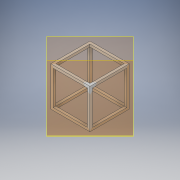
# Autodesk Inventor part: Outer
Saved by Autodesk Inventor 2019 (Build 230136000, 136)
## iProperties
Created: 2019-05-01
Part Number: Outer
Material: Generic
Document SubType Name: Modeling
Designer: Jorian Brusind
Density: 1 g/cm^3
Appearance: Default
Author: Jorian Brusind
Autodesk Inventor part; units mm, degrees
ref_plane "YZ Plane" through (0, 0, 0) normal (1, 0, 0) x (0, 1, 0)
ref_plane "XZ Plane" through (0, 0, 0) normal (0, 1, 0) x (-1, 0, 0)
ref_plane "XY Plane" through (0, 0, 0) normal (0, 0, 1) x (1, 0, 0)
sketch "Sketch1" plane through (0, 0, 0) normal (0, 1, 0) x (-1, 0, 0)
  line L0 (0, 0) -> (15, 0)
  line L1 (15, 0) -> (15, -15)
  line L2 (15, -15) -> (0, -15)
  line L3 (0, -15) -> (0, 0)
  dimension "d0" = 15
  dimension "d1" = 15
  constraints: 8 end point, 2 parallel, 1 horizontal, 1 perpendicular
  measures "d0" distance of L1.end L2.end
  measures "d1" distance of L0.end L1.end
extrude "Extrusion1" add sketch "Sketch1" along normal blind 15
sketch "Sketch2" plane through (0, 0, 0) normal (1, 0, 0) x (0, 0, -1)
  line L0 (15, 0) -> (0, 0) projected
  line L1 (0, 0) -> (1, 0)
  line L2 (1, 0) -> (1, 1)
  line L3 (1, 1) -> (14, 1)
  line L4 (14, 1) -> (14, 14)
  line L5 (14, 14) -> (1, 14)
  line L6 (1, 14) -> (1, 1)
  dimension "d4" = 1
  dimension "d5" = 1
  dimension "d6" = 13
  dimension "d7" = 13
  constraints: 12 end point, 2 parallel, 2 perpendicular, 1 horizontal, 1 point on line
  measures "d4" distance of L0.end L1.end
  measures "d5" distance of L1.end L2.end
  measures "d6" distance of L5.end L4.end
  measures "d7" distance of L4.end L3.end
extrude "Extrusion2" cut sketch "Sketch2" against normal blind 15
sketch "Sketch3" plane through (-15, 0, 0) normal (0, 0, 1) x (1, 0, 0)
  line L0 (0, 0) -> (0, 15) projected
  line L1 (0, 0) -> (1, 0)
  line L2 (15, 0) -> (0, 0) projected
  line L3 (1, 0) -> (1, 1)
  line L4 (1, 1) -> (14, 1)
  line L5 (14, 1) -> (14, 14)
  line L6 (14, 14) -> (1, 14)
  line L7 (1, 14) -> (1, 1)
  dimension "d10" = 1
  dimension "d11" = 1
  dimension "d12" = 13
  dimension "d13" = 13
  constraints: 12 end point, 2 parallel, 1 horizontal, 1 perpendicular, 1 point on line, 1 vertical
  measures "d10" distance of L0.start L1.end
  measures "d11" distance of L1.end L3.end
  measures "d12" distance of L6.end L5.end
  measures "d13" distance of L5.end L4.end
extrude "Extrusion3" cut sketch "Sketch3" against normal blind 15
sketch "Sketch4" plane through (0, 15, 0) normal (0, 1, 0) x (1, 0, 0)
  line L0 (-15, 0) -> (0, 0) projected
  line L1 (0, 0) -> (-1, 0)
  line L2 (-1, 0) -> (-1, 1)
  line L3 (-1, 0) -> (-1, 1) projected
  line L4 (-1, 1) -> (-14, 1)
  line L5 (-14, 1) -> (-14, 14)
  line L6 (-14, 14) -> (-1, 14)
  line L7 (-1, 14) -> (-1, 1)
  dimension "d16" = 1
  dimension "d17" = 1
  dimension "d18" = 13
  dimension "d19" = 13
  constraints: 12 end point, 2 parallel, 2 perpendicular, 1 horizontal, 1 point on line
  measures "d16" distance of L0.end L1.end
  measures "d17" distance of L1.end L2.end
  measures "d18" distance of L5.end L6.end
  measures "d19" distance of L4.end L5.end
extrude "Extrusion4" cut sketch "Sketch4" against normal blind 15
ref_plane "Work Plane2" through (-1, 14, -1) normal (0.5773503, 0.5773503, 0.5773503) x (-0.7071068, 0, 0.7071068)
ref_plane "Work Plane1" through (0, 15, -15) normal (0.5773503, 0.5773503, 0.5773503) x (-0.7071068, 0, 0.7071068)
sketch "Sketch5" plane through (-1, 14, -1) normal (0.5773503, 0.5773503, 0.5773503) x (-0.7071068, 0, 0.7071068)
  line L0 (0, 0) -> (-9.1924, -5.3072) projected
  circle A0 centre (0, 0) radius 0.5
  point P0 (0, 12.2474)
  dimension "d22" = 1
  constraints: 1 centre point
  measures "d22" diameter of A0
extrude "Extrusion5" add sketch "Sketch5" against normal blind 4
body "Solid1"
